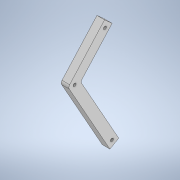
# Autodesk Inventor part: bogie1
Saved by Autodesk Inventor 2020 (Build 240168000, 168)
## iProperties
Created: 2020-05-20
Part Number: bogie1
Material: Generic
Document SubType Name: Modeling
Designer: Manish
Density: 1 g/cm^3
Appearance: Default
Author: Manish
Autodesk Inventor part; units mm, degrees
ref_plane "YZ Plane" through (0, 0, 0) normal (1, 0, 0) x (0, 1, 0)
ref_plane "XZ Plane" through (0, 0, 0) normal (0, 1, 0) x (-1, 0, 0)
ref_plane "XY Plane" through (0, 0, 0) normal (0, 0, 1) x (1, 0, 0)
sketch "Sketch1" plane through (0, 0, 0) normal (1, 0, 0) x (0, 1, 0)
  circle A0 centre (0, 0) radius 3
  line L0 (0, 0) -> (-4.9047, 8.7291)
  line L1 (-4.9047, 8.7291) -> (4.8923, -8.707)
  line L2 (-4.6236, -14.0538) -> (-134.5969, -87.0829)
  line L3 (-134.5969, -87.0829) -> (-144.3938, -69.6468)
  line L4 (-144.3938, -69.6468) -> (-1.8954, 10.42)
  line L5 (4.8923, -8.707) -> (13.6104, -3.8085)
  line L6 (13.6104, -3.8085) -> (3.8134, 13.6276)
  line L7 (3.8134, 13.6276) -> (-4.9047, 8.7291)
  line L8 (0, 0) -> (7.0679, 7.8353)
  line L9 (7.0679, 7.8353) -> (-6.3282, -7.0153)
  line L10 (2.3343, -14.8295) -> (67.9252, -73.9961)
  line L11 (67.9252, -73.9961) -> (81.3214, -59.1454)
  line L12 (81.3214, -59.1454) -> (7.0679, 7.8353)
  line L13 (-6.3282, -7.0153) -> (-13.7536, -0.3173)
  line L14 (-13.7536, -0.3173) -> (-0.3574, 14.5334)
  line L15 (5.0625, 9.6443) -> (7.0679, 7.8353)
  circle A1 centre (-133.3927, -74.9359) radius 3
  circle A2 centre (69.4256, -61.8821) radius 3
  arc A3 (5.0625, 9.6443) -> (-1.8954, 10.42) centre (1.0437, 5.1891) ccw
  arc A4 (2.3343, -14.8295) -> (-4.6236, -14.0538) centre (-1.6845, -19.2847) ccw
  point P0 (-161.0866, -23.1014)
  dimension "d0" = 20
  dimension "d1" = 160
  dimension "d2" = 20
  dimension "d3" = 10
  dimension "d4" = 20
  dimension "d5" = 100
  dimension "d6" = 10
  dimension "d7" = 20
  dimension "d8" = 6
  dimension "d9" = 6
  dimension "d10" = 6
  dimension "d11" = 6
  dimension "d14" = 7
  dimension "d15" = 7
  dimension "d16" = 10
  dimension "d17" = 10
  dimension "d27" = 108.617
  dimension "d28" = 9.9873
  dimension "d29" = 204.1388
  dimension "d30" = 115.6029
  constraints: 32 end point, 10 point on line, 7 coincident, 6 perpendicular, 5 centre point, 4 point on circle, 4 tangent, 1 collinear, 1 equal radius
  measures "d0" distance of L1.start L1.end
  measures "d1" distance of L1.end L3.start
  measures "d2" distance of L3.start L4.start
  measures "d3" distance of L1.end L6.start
  measures "d4" distance of L8.end L13.start
  measures "d5" distance of L13.start L11.start
  measures "d6" distance of L13.start L13.end
  measures "d7" distance of L13.end L14.end
  measures "d8" diameter of A1
  measures "d9" diameter of A2
  measures "d10" radius of A3
  measures "d11" radius of A4
  measures "d14" distance from line of point (69.426, -61.882) L11
  measures "d15" distance from line of A1.centre L3
  measures "d16" distance from line of point (-133.393, -74.936) L4
  measures "d17" distance from line of point (69.426, -61.882) L10
  measures "d27" angle of L2 L10
  measures "d28" distance from line of point (0, 0) L5
  measures "d29" distance from line of point (-161.087, -23.101) L11
  measures "d30" distance from line of point (-161.087, -23.101) L10
extrude "Extrusion1" add sketch "Sketch1" along normal blind 15 contours A0 L1 L8 | A0 L8 L6 L5 L1 | L8 L0 A0 | A0 L0 L4 A3 L15 L8 | L1 L5 L6 L12 L11 L10 A4 L2 L3 L4 L14 L13 L9 A0 | A0 L9 L1 | L0 L9 A0 | A0 L9 L13 L14 L4 L0 | A1 | A2
sketch "Sketch2" plane through (0, 0, 0) normal (-1, 0, 0) x (0, 0, 1)
  circle A0 centre (0, 0) radius 3
  circle A1 centre (-59.8727, 67.1979) radius 3
  line L0 (-73.9961, 67.9252) -> (-59.1454, 81.3214) projected
  line L1 (-14.8295, 2.3343) -> (-73.9961, 67.9252) projected
  circle A2 centre (-73.4663, -130.7773) radius 3
  line L2 (10.42, -1.8954) -> (-69.6468, -144.3938) projected
  line L3 (-69.6468, -144.3938) -> (-87.0829, -134.5969) projected
  dimension "d18" = 6
  dimension "d19" = 6
  dimension "d20" = 10
  dimension "d21" = 10
  dimension "d22" = 6
  dimension "d23" = 10
  dimension "d24" = 10
  constraints: 3 centre point, 1 coincident
  measures "d18" diameter of A0
  measures "d19" diameter of A1
  measures "d20" distance from line of A1.centre L0
  measures "d21" distance from line of A1.centre L1
  measures "d22" diameter of A2
  measures "d23" distance from line of L2 A2.centre
  measures "d24" distance from line of L3 A2.centre
extrude "Extrusion2" cut sketch "Sketch2" against normal through all
body "Solid1"
